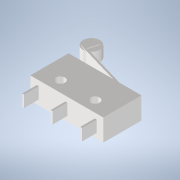
# Autodesk Inventor part: 00_Endstop_mechanical_vuniversum_microswitch_roll
Saved by Autodesk Inventor 2022 (Build 260153000, 153)
## iProperties
Created: 2022-10-23
Part Number: 00_Endstop_mechanical_vuniversum_microswitch_roll
Material: Generisch
Document SubType Name: Modeling
Designer: diederichbenedict
Density: 1 g/cm^3
Appearance: Vorgabe
Author: diederichbenedict
Autodesk Inventor part; units mm, degrees
ref_plane "YZ Plane" through (0, 0, 0) normal (1, 0, 0) x (0, 1, 0)
ref_plane "XZ Plane" through (0, 0, 0) normal (0, 1, 0) x (-1, 0, 0)
ref_plane "XY Plane" through (0, 0, 0) normal (0, 0, 1) x (1, 0, 0)
sketch "Skizze1" plane through (0, 0, 0) normal (0, 1, 0) x (-1, 0, 0)
  line L0 (-10, -5.25) -> (10, -5.25)
  line L1 (10, -5.25) -> (10, 5.25)
  line L2 (10, 5.25) -> (-10, 5.25)
  line L3 (-10, 5.25) -> (-10, -5.25)
  line L4 (-10, -5.25) -> (10, 5.25) construction
  line L5 (10, -5.25) -> (-10, 5.25) construction
  circle A0 centre (4.75, 2.25) radius 1.25
  circle A1 centre (-4.75, 2.25) radius 1.25
  point P0 (0, 0)
  dimension "d0" = 20
  dimension "d1" = 10.5
  dimension "d4" = 2.5
  dimension "d5" = 2.5
  dimension "d6" = 4.75
  dimension "d7" = 3
  dimension "d8" = 3
  dimension "d9" = 4.75
  constraints: 12 end point, 2 centre point, 2 midpoint, 2 parallel, 1 horizontal, 1 perpendicular
  measures "d0" distance of L2.end L1.end
  measures "d1" distance of L1.end L0.end
  measures "d4" diameter of A0
  measures "d5" diameter of A1
  measures "d6" horizontal distance of A0.centre point (0, 0)
  measures "d7" distance from line of A0.centre L2
  measures "d8" distance from line of L2 A1.centre
  measures "d9" horizontal distance of A1.centre point (0, 0)
extrude "Extrusion1" add sketch "Skizze1" along normal mid plane 6
sketch "Skizze2" plane through (0, 0, 0) normal (0, 1, 0) x (-1, 0, 0)
  line L0 (10, -5.25) -> (10, 5.25) projected
  line L1 (10, 5.25) -> (-10, 5.25) projected
  line L2 (-10, 5.25) -> (-10, -5.25) projected
  line L3 (-10, -5.25) -> (10, -5.25) projected
  circle A0 centre (4.75, 2.25) radius 1.25 projected
  circle A1 centre (-4.75, 2.25) radius 1.25 projected
  line L4 (10, 5.25) -> (-10, 5.25) projected
  line L5 (8.2, 5.25) -> (7.7, 5.25)
  line L6 (7.7, 5.25) -> (7.7, 9.25)
  line L7 (7.7, 9.25) -> (8.2, 9.25)
  line L8 (8.2, 9.25) -> (8.2, 5.25)
  line L9 (0.3746, 5.25) -> (-0.1254, 5.25)
  line L10 (-0.1254, 5.25) -> (-0.1254, 9.25)
  line L11 (-0.1254, 9.25) -> (0.3746, 9.25)
  line L12 (0.3746, 9.25) -> (0.3746, 5.25)
  line L13 (-7.7, 5.25) -> (-8.2, 5.25)
  line L14 (-8.2, 5.25) -> (-8.2, 9.25)
  line L15 (-8.2, 9.25) -> (-7.7, 9.25)
  line L16 (-7.7, 9.25) -> (-7.7, 5.25)
  point P0 (0, 0)
  dimension "d10" = 0.5
  dimension "d11" = 4
  dimension "d12" = 1.8
  dimension "d13" = 1.8
  dimension "d14" = 0.5
  dimension "d15" = 0.5
  constraints: 24 end point, 6 parallel, 5 point on line, 3 horizontal, 3 perpendicular
  measures "d10" distance of L6.end L7.end
  measures "d11" distance of L5.end L6.end
  measures "d12" distance between parallel lines of L14 L2
  measures "d13" distance between parallel lines of L8 L0
  measures "d14" distance between parallel lines of L14 L16
  measures "d15" distance between parallel lines of L10 L12
extrude "Extrusion2" add sketch "Skizze2" along normal mid plane 3.2 contours L1 L6 L7 L8 | L14 L15 L16 L1 | L1 L10 L11 L12
sketch "Skizze3" plane through (0, 0, 0) normal (0, 1, 0) x (-1, 0, 0)
  line L0 (10, -5.25) -> (10, 5.25) projected
  line L1 (10, 5.25) -> (-10, 5.25) projected
  line L2 (-10, 5.25) -> (-10, -5.25) projected
  line L3 (-10, -5.25) -> (10, -5.25) projected
  circle A0 centre (4.75, 2.25) radius 1.25 projected
  circle A1 centre (-4.75, 2.25) radius 1.25 projected
  line L4 (10, -5.25) -> (-10, -5.25) projected
  line L5 (-7.1, -5.25) -> (9.9766, -10.265)
  line L6 (9.9766, -10.265) -> (9.1627, -13.0362)
  line L7 (9.1627, -13.0362) -> (10.7453, -13.501)
  line L8 (10.7453, -13.501) -> (11.7, -10.25)
  line L9 (11.7, -10.25) -> (-5.3255, -5.25)
  point P0 (0, 0)
  dimension "d18" = 2.9
  dimension "d19" = 0.5
  dimension "d20" = 1.7
  dimension "d21" = 5
  constraints: 10 end point, 3 parallel, 2 point on line, 1 perpendicular
  measures "d18" distance from line of L5.start L2
  measures "d19" distance between parallel lines of L5 L9
  measures "d20" distance from line of L0 L8.end
  measures "d21" distance from line of L8.end L3
extrude "Extrusion3" add sketch "Skizze3" along normal mid plane 3.4 contours L9 L8 L7 L6 L5 L3
sketch "Skizze4" plane through (0, 0, 0) normal (0, 1, 0) x (-1, 0, 0)
  line L0 (11.7, -10.25) -> (-5.3255, -5.25) projected
  line L1 (-7.1, -5.25) -> (-5.3255, -5.25) projected
  line L2 (-7.1, -5.25) -> (9.9766, -10.265) projected
  line L3 (9.9766, -10.265) -> (9.1627, -13.0362) projected
  line L4 (9.1627, -13.0362) -> (10.7453, -13.501) projected
  line L5 (10.7453, -13.501) -> (11.7, -10.25) projected
  circle A0 centre (10.3631, -11.8755) radius 2.3
  point P0 (0, 0)
  dimension "d24" = 4.6
  constraints: 1 centre point
  measures "d24" diameter of A0
extrude "Extrusion4" add sketch "Skizze4" along normal mid plane 3 contours L5 L4 L3 L2 A0 L0 | L0 A0 L2 L3 L4 L5
